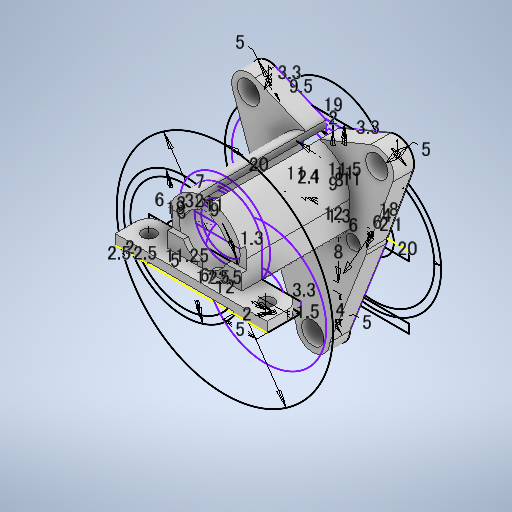
# Autodesk Inventor part: ikafly2a
Saved by Autodesk Inventor 2025 (Build 290162000, 162)
## iProperties
Created: 2024-06-09
Part Number: ikafly2a
Material: 一般
Document SubType Name: Modeling
Designer: Saigusa
Density: 1 g/cm^3
Appearance: 既定
Author: Saigusa
Autodesk Inventor part; units mm, degrees
ref_plane "YZ Plane" through (0, 0, 0) normal (1, 0, 0) x (0, 1, 0)
ref_plane "XZ Plane" through (0, 0, 0) normal (0, 1, 0) x (-1, 0, 0)
ref_plane "XY Plane" through (0, 0, 0) normal (0, 0, 1) x (1, 0, 0)
sketch "スケッチ1" plane through (0, 0, 0) normal (0, 0, 1) x (1, 0, 0)
  circle A0 centre (0, 0) radius 16
  line L0 (0, 0) -> (-6, 0)
  line L1 (-6, 0) -> (6, 0)
  circle A1 centre (-6, 0) radius 9
  circle A2 centre (-6, 0) radius 3
  circle A3 centre (6, 0) radius 9
  circle A4 centre (6, 0) radius 3
  circle A5 centre (-6, 0) radius 8
  circle A6 centre (0, 5.2915) radius 5
  circle A7 centre (0, 5.2915) radius 4.5
  circle A8 centre (0, 5.2915) radius 5.5
  circle A9 centre (0, 5.2915) radius 3.5
  line L2 (0, 0) -> (-11.25, 0)
  line L3 (-11.25, 0) -> (11.25, 0)
  line L4 (-11.25, 0) -> (11.25, 0)
  line L5 (11.25, 0) -> (11.25, 1.5)
  line L6 (11.25, 1.5) -> (-11.25, 1.5)
  line L7 (-11.25, 1.5) -> (-11.25, 0)
  line L8 (0, 5.2915) -> (-5.5, 5.2915)
  line L9 (0, 5.2915) -> (5.5, 5.2915)
  line L10 (5.5, 3.7915) -> (-5.5, 3.7915)
  line L11 (-5.5, 3.7915) -> (-5.5, 6.7915)
  line L12 (-5.5, 6.7915) -> (5.5, 6.7915)
  line L13 (5.5, 6.7915) -> (5.5, 3.7915)
  line L14 (5.5, 3.7915) -> (-5.5, 6.7915) construction
  line L15 (-5.5, 3.7915) -> (5.5, 6.7915) construction
  line L16 (-5.5, 5.2915) -> (-5.5, 1.5)
  line L17 (5.5, 5.2915) -> (5.5, 1.5)
  line L18 (5.2915, 3.7915) -> (5.2915, 1.5)
  line L19 (-5.2915, 3.7915) -> (-5.2915, 1.5)
  circle A10 centre (0, 5.2915) radius 6.6802
  point P0 (-3.9843, 1.5)
  point P1 (3.9843, 1.5)
  point P2 (4.0774, 0)
  point P3 (1.5, 0)
  point P4 (-4.0774, 0)
  point P5 (-1.5, 0)
  dimension "d0" = 32
  dimension "d1" = 6
  dimension "d2" = 12
  dimension "d3" = 18
  dimension "d4" = 6
  dimension "d5" = 16
  dimension "d6" = 9
  dimension "d7" = 11
  dimension "d8" = 7
  dimension "d9" = 11.25
  dimension "d10" = 22.5
  dimension "d11" = 1.5
  dimension "d12" = 3
  constraints: 40 end point, 11 point on line, 10 centre point, 10 coincident, 6 point on circle, 5 perpendicular, 4 horizontal, 4 parallel, 2 midpoint, 1 tangent, 3 other
  measures "d0" diameter of A0
  measures "d1" distance of L0.start L0.end
  measures "d2" distance of L0.end L1.end
  measures "d3" diameter of A1
  measures "d4" diameter of A2
  measures "d5" diameter of A5
  measures "d6" diameter of A7
  measures "d7" diameter of A8
  measures "d8" diameter of A9
  measures "d9" distance of L0.start L2.end
  measures "d10" distance of L2.end L3.end
  measures "d11" distance of L5.end L4.end
  measures "d12" distance of L10.end L11.end
extrude "押し出し1" add sketch "スケッチ1" along normal blind 5 contours L0 A8 A3 A6 A5 L1 | L0 A3 A8 | A8 A5 L1 | L0 A10 L6 A8 A2 | A2 A8 A3 | A8 A2 L6 A6 A3 | A5 A8 A1 L1 | A5 A6 A1 A8 | L0 L2 A2 L6 A10 | A8 L6 A2 | A6 L6 A3 | A3 L6 A7 A5 A6 | A4 A8 L6 A10 L1 | A1 A8 A4 | A5 A7 L6 A1 A6 | A1 A6 L6 A4 A8 | L2 L7 L6 A2 | A10 L6 A4 L3 L1 | A4 L6 A8 | A7 L6 A5 | A5 L6 A7 | A1 L6 A6 | A4 L6 L5 L3 picked at (2.524, 0.7859) picked at (-3.6973, 1.4091) picked at (3.6973, 1.4091)
extrude "押し出し2" add sketch "スケッチ1" along normal blind 3 contours L0 A8 A3 A6 A5 L1 | A8 A2 L6 A6 A3 | A5 A6 A1 A8 | A8 L6 A2 | A6 L6 A3 | A3 L6 A7 A5 A6 | A5 A7 L6 A1 A6 | A1 A6 L6 A4 A8 | L16 A2 L19 L6 | L6 A8 A2 | A2 A6 L6 | L6 L19 A2 A8 | L6 A6 L10 A7 A3 | A3 A7 L6 | A4 L6 A8 | A7 L6 A5 | A5 L6 A7 | A1 L6 A6 | L16 L10 L19 A2 | A2 A8 L10 A6 | A2 L19 A8 | A7 L10 A9 A3 | A3 A9 A5 L6 A7 | L6 L18 A4 L17 | L6 A6 A4 | A4 A8 L6 | A8 A4 L18 L6 | A5 A9 A1 A7 L6 | A7 A1 L6 | A1 A7 L10 A6 L6 | L11 A8 L10 | L10 A8 L8 A6 | A6 L8 A7 L10 | A8 A1 A6 A5 | A5 A6 L12 A8 | A7 L8 A9 L10 | A4 L18 L10 L17 | A6 L10 A8 A4 | A8 L18 A4 | A1 A9 L10 A7 | A8 L12 A6 L8 | A6 L12 A7 L8 | A8 A3 A6 A1 | A6 A1 A7 A5 | A5 A7 L12 A6 | A7 L12 A9 L8 | L10 A8 L13 | L10 A7 L9 A6 | A6 L9 A8 L10 | L10 A9 L9 A7 | A6 A3 A7 A1 | A8 L12 A6 A3 | A7 A1 A9 A5 | A5 A9 L12 A7 | L9 A6 L12 A8 | L9 A7 L12 A6 | L9 A9 L12 A7 | A7 A3 A9 A1 | A6 L12 A7 A3 | L12 A9 A3 A7
extrude "押し出し3" cut sketch "スケッチ1" along normal blind 2.25 contours A7 L6 A5 | A5 L6 A7 | A7 L10 A9 A3 | A3 A9 A5 L6 A7 | A5 A9 A1 A7 L6 | A7 L8 A9 L10 | A1 A9 L10 A7 | A7 L12 A9 L8 | L10 A9 L9 A7 | A7 A1 A9 A5 | A5 A9 L12 A7 | L9 A9 L12 A7 | A7 A3 A9 A1 | L12 A9 A3 A7
sketch "スケッチ2" plane through (0, 0, 3) normal (0, 0, 1) x (1, 0, 0)
  line L0 (5.5, 3.7903) -> (-5.5, 3.7903)
  line L1 (-5.5, 3.7903) -> (-5.5, 6.7903)
  line L2 (-5.5, 6.7903) -> (5.5, 6.7903)
  line L3 (5.5, 6.7903) -> (5.5, 3.7903)
  line L4 (5.5, 3.7903) -> (-5.5, 6.7903) construction
  line L5 (-5.5, 3.7903) -> (5.5, 6.7903) construction
  point P0 (0, 0)
  point P1 (0, 5.2903)
  dimension "d19" = 11
  dimension "d20" = 3
  constraints: 12 end point, 2 midpoint, 2 parallel, 1 horizontal, 1 perpendicular
  measures "d19" distance of L1.end L2.end
  measures "d20" distance of L0.end L1.end
extrude "押し出し4" cut sketch "スケッチ2" against normal blind 0.75
extrude "押し出し5" add sketch "スケッチ1" against normal blind 16 contours L1 A8 L0 | L0 A8 A3 A6 A5 L1 | L0 A3 A8 | A8 A5 L1 | L0 A10 L6 A8 A2 | A2 A8 A3 | A8 A2 L6 A6 A3 | A5 A8 A1 L1 | A5 A6 A1 A8 | A8 L6 A2 | A6 L6 A3 | A3 L6 A7 A5 A6 | A4 A8 L6 A10 L1 | A1 A8 A4 | A5 A7 L6 A1 A6 | A1 A6 L6 A4 A8 | L16 A2 L19 L6 | L6 A8 A2 | A2 A6 L6 | L6 L19 A2 A8 | L6 A6 L10 A7 A3 | A3 A7 L6 | A4 L6 A8 | A1 L6 A6 | L16 L10 L19 A2 | A2 A8 L10 A6 | A2 L19 A8 | L6 L18 A4 L17 | L6 A6 A4 | A4 A8 L6 | A8 A4 L18 L6 | A7 A1 L6 | A1 A7 L10 A6 L6 | L11 A8 L10 | L10 A8 L8 A6 | A6 L8 A7 L10 | A8 A1 A6 A5 | A5 A6 L12 A8 | A4 L18 L10 L17 | A6 L10 A8 A4 | A8 L18 A4 | A8 L12 A6 L8 | A6 L12 A7 L8 | A8 A3 A6 A1 | A6 A1 A7 A5 | A5 A7 L12 A6 | L10 A8 L13 | L10 A7 L9 A6 | A6 L9 A8 L10 | A6 A3 A7 A1 | A8 L12 A6 A3 | L9 A6 L12 A8 | L9 A7 L12 A6 | A6 L12 A7 A3
sketch "電池" plane through (0, 0, -16) normal (0, 0, -1) x (-1, 0, 0)
  line L0 (0, 0) -> (0, 8)
  circle A0 centre (0, 8) radius 8
  dimension "d34" = 8
  constraints: 2 end point, 1 coincident, 1 vertical, 1 vertical alignment, 2 other
  measures "d34" distance of L0.start L0.end
sketch "スケッチ3" plane through (0, 5.2915, -16) normal (0, 0, -1) x (-1, 0, 0)
  line L0 (0, -5.2915) -> (-6, -5.2915)
  line L1 (11.25, -5.2915) -> (-11.25, -5.2915) projected
  line L2 (-6, -5.2915) -> (6, -5.2915)
  circle A0 centre (-6, -5.2915) radius 3
  circle A1 centre (-6, -5.2915) radius 9
  circle A2 centre (6, -5.2915) radius 3
  circle A3 centre (6, -5.2915) radius 9
  circle A4 centre (-6, -5.2915) radius 10
  circle A5 centre (6, -5.2915) radius 10
  line L3 (0, -5.2915) -> (11, -5.2915)
  line L4 (0, -5.2915) -> (0, 6.2085)
  line L5 (0, 6.2085) -> (9.5, 6.2085)
  line L6 (9.5, 6.2085) -> (-9.5, 6.2085)
  circle A6 centre (-9.5, 6.2085) radius 1.65
  circle A7 centre (9.5, 6.2085) radius 1.65
  circle A8 centre (-9.5, 6.2085) radius 2.5
  circle A9 centre (9.5, 6.2085) radius 2.5
  circle A10 centre (6, -5.2915) radius 1.05
  circle A11 centre (-6, -5.2915) radius 1.05
  line L7 (0, -5.2915) -> (0, -6.5915)
  line L8 (-5.5, -3.7915) -> (-5.5, -1.5012) projected
  line L9 (0, -6.5915) -> (11.25, -6.5915)
  line L10 (11.25, -6.5915) -> (11.25, -5.2915)
  line L11 (0, -6.5915) -> (-11.25, -6.5915)
  line L12 (-11.25, -6.5915) -> (-11.25, -5.2915)
  line L13 (0, -6.5915) -> (0, -14.5915)
  line L14 (0, -14.5915) -> (11.25, -14.5915)
  line L15 (11.25, -14.5915) -> (11.25, -15.8915)
  line L16 (11.25, -15.8915) -> (-11.25, -15.8915)
  line L17 (-11.25, -15.8915) -> (-11.25, -14.5915)
  line L18 (0, -14.5915) -> (-11.25, -14.5915)
  line L19 (0, -15.8915) -> (0, -19.8915)
  circle A12 centre (0, -19.8915) radius 1.65
  circle A13 centre (0, -19.8915) radius 2.5
  line L20 (-2.5, -19.8915) -> (2.5, -19.8915)
  circle A14 centre (0, 0) radius 5.5
  circle A15 centre (-6, -5.2915) radius 2
  circle A16 centre (6, -5.2915) radius 2
  line L21 (-9.5, 3.7085) -> (9.5, 3.7085)
  line L22 (-8, -5.2915) -> (-8, 3.7085)
  line L23 (8, -5.2915) -> (8, 3.7085)
  line L24 (-6, -7.2915) -> (6, -7.2915)
  line L25 (2.5, -19.8915) -> (2.5, -7.2915)
  line L26 (-2.5, -19.8915) -> (-2.5, -7.2915)
  line L27 (1, -5.5) -> (-1, -5.5)
  line L28 (-1, -5.5) -> (-1, 5.5)
  line L29 (-1, 5.5) -> (1, 5.5)
  line L30 (1, 5.5) -> (1, -5.5)
  line L31 (1, -5.5) -> (-1, 5.5) construction
  line L32 (-1, -5.5) -> (1, 5.5) construction
  circle A17 centre (0, 0) radius 4.5
  line L33 (-1, 5.4083) -> (-8.5471, 8.5198)
  line L34 (1, 5.4083) -> (8.5471, 8.5198)
  line L35 (-8, -5.2915) -> (-11.851, 5.3584)
  line L36 (8, -5.2915) -> (11.851, 5.3584)
  line L37 (-2.5, -19.8915) -> (-7.8655, -6.0127)
  line L38 (2.5, -19.8915) -> (7.8655, -6.0127)
  point P0 (3.7639, -7.2915)
  point P1 (3.798, -7.2915)
  point P2 (3.7917, -7.3221)
  point P3 (-3.7639, -7.2915)
  point P4 (-3.7917, -7.3221)
  point P5 (-3.798, -7.2915)
  point P6 (3, -5.2915)
  point P7 (1.5, -5.2915)
  point P8 (-1.5, -5.2915)
  point P9 (-4, -5.2915)
  point P10 (-3.8997, -3.8785)
  point P11 (3.0937, -4.5474)
  point P12 (-1, -4.3875)
  point P13 (1, -4.3875)
  point P14 (1, 5.4083)
  dimension "d25" = 6
  dimension "d26" = 12
  dimension "d27" = 6
  dimension "d28" = 18
  dimension "d35" = 20
  dimension "d36" = 20
  dimension "d37" = 11
  dimension "d38" = 11.5
  dimension "d39" = 9.5
  dimension "d40" = 19
  dimension "d41" = 3.3
  dimension "d42" = 3.3
  dimension "d43" = 5
  dimension "d44" = 5
  dimension "d45" = 2.1
  dimension "d46" = 2.1
  dimension "d47" = 1.3
  dimension "d48" = 8
  dimension "d49" = 1.3
  dimension "d50" = 4
  dimension "d51" = 3.3
  dimension "d52" = 5
  dimension "d53" = 11
  dimension "d54" = 4
  dimension "d55" = 4
  dimension "d56" = 2
  dimension "d57" = 11
  dimension "d58" = 9
  constraints: 74 end point, 19 point on line, 18 centre point, 17 coincident, 17 point on circle, 12 perpendicular, 11 tangent, 3 midpoint, 3 parallel, 2 horizontal, 1 vertical
  measures "d25" distance of L0.start L0.end
  measures "d26" distance of L0.end L2.end
  measures "d27" diameter of A0
  measures "d28" diameter of A1
  measures "d35" diameter of A4
  measures "d36" diameter of A5
  measures "d37" distance of L0.start L3.end
  measures "d38" distance of L0.start L4.end
  measures "d39" distance of L4.end L5.end
  measures "d40" distance of L5.end L6.end
  measures "d41" diameter of A6
  measures "d42" diameter of A7
  measures "d43" diameter of A8
  measures "d44" diameter of A9
  measures "d45" diameter of A10
  measures "d46" diameter of A11
  measures "d47" distance of L0.start L7.end
  measures "d48" distance of L7.end L13.end
  measures "d49" distance of L14.end L15.end
  measures "d50" distance of L19.start L19.end
  measures "d51" diameter of A12
  measures "d52" diameter of A13
  measures "d53" diameter of A14
  measures "d54" diameter of A15
  measures "d55" diameter of A16
  measures "d56" distance of L28.end L29.end
  measures "d57" distance of L27.end L28.end
  measures "d58" diameter of A17
sketch "スケッチ4" plane through (-11.25, 0, 5) normal (0, -1, 0) x (1, 0, 0)
  line L0 (0, 0) -> (22.5, 0) projected
  line L1 (0, 0) -> (2.5, 0)
  line L2 (2.5, 0) -> (2.5, -2.5)
  line L3 (2.5, -2.5) -> (20, -2.5)
  circle A0 centre (2.5, -2.5) radius 1
  circle A1 centre (20, -2.5) radius 1
  line L4 (0.1664, -5) -> (4.8336, -5)
  line L5 (4.8336, -5) -> (4.8336, 0)
  line L6 (4.8336, 0) -> (0.1664, 0)
  line L7 (0.1664, 0) -> (0.1664, -5)
  line L8 (0.1664, -5) -> (4.8336, 0) construction
  line L9 (4.8336, -5) -> (0.1664, 0) construction
  line L10 (22.5, -5) -> (17.5, -5)
  line L11 (17.5, -5) -> (17.5, 0)
  line L12 (17.5, 0) -> (22.5, 0)
  line L13 (22.5, 0) -> (22.5, -5)
  line L14 (22.5, -5) -> (17.5, 0) construction
  line L15 (17.5, -5) -> (22.5, 0) construction
  line L16 (4.8336, -5) -> (17.5, -5)
  point P0 (11.25, -5)
  dimension "d29" = 2.5
  dimension "d30" = 2.5
  dimension "d31" = 17.5
  dimension "d32" = 2
  dimension "d33" = 2
  dimension "d63" = 5
  dimension "d64" = 5
  constraints: 32 end point, 4 midpoint, 4 parallel, 4 perpendicular, 2 centre point, 2 coincident, 2 horizontal, 2 point on line
  measures "d29" distance of L0.start L1.end
  measures "d30" distance of L1.end L2.end
  measures "d31" distance of L2.end L3.end
  measures "d32" diameter of A0
  measures "d33" diameter of A1
  measures "d63" distance of L5.end L4.end
  measures "d64" distance of L11.end L12.end
extrude "押し出し6" add sketch "スケッチ3" against normal blind 3 contours A0 L11 A5 L0 | A3 L11 A0 | L0 A14 L28 L27 L7 L11 A3 | A15 L11 L1 A11 L0 | A15 L8 A0 A14 A5 | L0 A11 L1 A15 | A5 L11 A15 | L11 A3 L24 A0 | A0 L24 A5 L11 | L11 L13 L24 A3 | A5 L24 A15 L11 | A15 L22 A0 L8 | A15 L11 | A14 L27 L28 | L24 A3 L26 A5 A0 | L24 L26 A3 | L7 L27 L30 A14 L1 A1 L9 | L9 A1 L24 L13 | A0 L22 A1 A14 | A5 A0 L37 L11 A15 L24 | L35 A0 L22 | L11 L37 A15 | A14 L30 L27 | A5 L26 A1 L37 A0 | L26 L24 L13 A3 | A3 A1 A5 L26 | L9 A2 L24 A1 | A1 A2 L9 | L24 L25 A1 L13 | A1 L21 A14 | A0 L35 A1 L22 | A5 A1 L26 | L13 A5 A1 | A1 L25 A4 A3 | A3 A4 L13 | L24 A2 A4 L25 A1 | A1 L25 L24 | A2 A14 A4 L1 | L1 A4 L9 A2 | L9 A4 L24 A2 | A1 L22 L21 | L21 A8 A4 A14 | A1 L35 A4 A8 L21 L22 | A1 L26 L18 L37 | A5 A4 L18 L26 A1 | A4 L25 A3 | A3 L25 L14 A5 A4 | L13 L18 A4 | A5 L14 L13 | A16 L1 A10 | A16 L9 A4 | A4 A14 A2 L23 A16 | L1 A10 A16 L9 | L9 A16 L24 A4 | A4 A8 L6 L33 A14 | L35 A8 A4 | L18 L26 A4 L37 | L18 A4 L26 | A4 A2 L38 A3 L25 | A3 L38 L14 L25 | L18 L14 A5 L25 L16 L26 A4 | L14 L25 A5 | A4 L24 A16 L9 L38 A2 | L23 A2 L36 | L9 A16 | A8 A4 | A4 A8 | A4 L26 L16 L37 | L14 L38 A5 L25 | A5 L38 L16 L25 | A14 A3 L23 A2 | L38 L9 A16 | L23 A3 L36 A2 | A8 L33 L6 | L16 L26 L37 | L16 L19 A13 L26 | A14 L21 A3 | L25 A13 L19 L16 | L16 L38 L25 | L23 L21 A9 A5 L36 A3 | A3 L21 L23 | L34 L5 A9 A5 A14 | L20 A12 A13 | A13 L19 A12 L20 | L21 A14 A5 A9 | L20 A12 L19 A13 | A5 A9 L36 | L34 A9 L5 | A9 A5 | A5 A9
extrude "押し出し7" cut sketch "スケッチ3" against normal blind 19 contours L28 A3 L4 A17 | L28 A5 A1 A3 | L4 A1 L30 A17 | L28 A1 A5 | A3 A4 L30 A1 | L4 A4 A3 | A1 A5 L4 | A1 L28 A4 A5 | A4 A5 L30 A3 | A3 L30 A4 | L4 L21 L30 A5 | A4 L28 L21 L4 | L21 L28 A17 L4 | L4 A17 L30 L21 | A14 L4 A17 L28 | L4 A14 L30 A17
extrude "押し出し8" cut sketch "スケッチ4" against normal blind 0.3 contours L0 L11 L3 L5 | L5 L3 L11 L16
extrude "押し出し9" cut sketch "スケッチ4" against normal blind 1.5 contours A0 L3 L2 | L2 L3 A0 | A1
fillet "フィレット1" radius 2 2 edges at (-11.25, 0.75, 0) (11.25, 0.75, 0)
